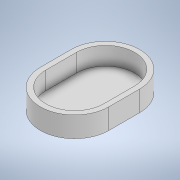
# Autodesk Inventor part: Riel2
Saved by Autodesk Inventor 2021 (Build 250183000, 183)
## iProperties
Created: 2021-06-11
Part Number: Riel2
Material: Genérico
Document SubType Name: Modeling
Designer: Mecatronica
Density: 1 g/cm^3
Appearance: Valor por defecto
Author: Mecatronica
Autodesk Inventor part; units mm, degrees
ref_plane "YZ Plane" through (0, 0, 0) normal (1, 0, 0) x (0, 1, 0)
ref_plane "XZ Plane" through (0, 0, 0) normal (0, 1, 0) x (-1, 0, 0)
ref_plane "XY Plane" through (0, 0, 0) normal (0, 0, 1) x (1, 0, 0)
sketch "Boceto1" plane through (0, 0, 0) normal (0, 1, 0) x (-1, 0, 0)
  line L0 (66.6667, 30) -> (-66.6667, 30)
  line L1 (-66.6667, 30) -> (-66.6667, -30)
  line L2 (-66.6667, -30) -> (66.6667, -30)
  line L3 (66.6667, -30) -> (66.6667, 30)
  arc A0 (66.6667, 30) -> (-66.6667, 30) centre (0, 30) ccw
  arc A1 (-66.6667, -30) -> (66.6667, -30) centre (0, -30) ccw
  point P0 (0, 0)
  dimension "d0" = 60
  dimension "d1" = 30
  dimension "d2" = 133.3333
  constraints: 8 end point, 4 point on circle, 4 tangent, 2 centre point, 2 parallel, 1 horizontal, 1 perpendicular
  measures "d0" distance of L0.end L1.end
  measures "d1" distance from line of L2 point (0, 0)
  measures "d2" distance of L0.start L0.end
extrude "Extrusión1" add sketch "Boceto1" along normal blind 40
sketch "Boceto2" plane through (0, 40, 0) normal (0, 1, 0) x (1, 0, 0)
  line L0 (-56.6667, -29.6296) -> (56.6667, -29.6296)
  line L1 (56.6667, -29.6296) -> (56.6667, 30.3704)
  line L2 (56.6667, 30.3704) -> (-56.6667, 30.3704)
  line L3 (-56.6667, 30.3704) -> (-56.6667, -29.6296)
  line L4 (66.6667, -30) -> (66.6667, 30) projected
  arc A0 (66.6667, 30) -> (-66.6667, 30) centre (0, 30) ccw projected
  line L5 (-66.6667, 30) -> (-66.6667, -30) projected
  arc A1 (-66.6667, -30) -> (66.6667, -30) centre (0, -30) ccw projected
  arc A2 (-56.6667, -29.6296) -> (56.6667, -29.6296) centre (0, -29.6296) ccw
  arc A3 (56.6667, 30.3704) -> (-56.6667, 30.3704) centre (0, 30.3704) ccw
  point P0 (0, 0)
  dimension "d5" = 60
  dimension "d6" = 10
  dimension "d7" = 10
  constraints: 8 end point, 4 point on circle, 4 tangent, 2 centre point, 2 parallel, 1 horizontal, 1 perpendicular
  measures "d5" distance of L2.end L0.start
  measures "d6" distance between parallel lines of L3 L5
  measures "d7" distance between parallel lines of L4 L1
extrude "Extrusión2" cut sketch "Boceto2" against normal blind 35 contours L3 L2 L1 L0 | L0 A2 | A3 L2
equation "\"d1\" = 0.5 * d0"
